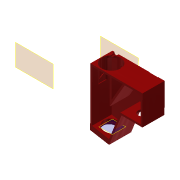
# Autodesk Inventor part: cellSTORM_v5_opticalstage
Saved by Autodesk Inventor 2022 (Build 260153000, 153)
## iProperties
Created: 2020-04-25
Part Number: cellSTORM_v5_opticalstage
Material: Generic
Document SubType Name: Modeling
Designer: diederichbenedict
Density: 1 g/cm^3
Appearance: Red
Author: diederichbenedict
Autodesk Inventor part; units mm, degrees
ref_plane "YZ Plane" through (0, 0, 0) normal (1, 0, 0) x (0, 1, 0)
ref_plane "XZ Plane" through (0, 0, 0) normal (0, 1, 0) x (-1, 0, 0)
ref_plane "XY Plane" through (0, 0, 0) normal (0, 0, 1) x (1, 0, 0)
ref_plane "Work Plane1" through (0, 0, 0) normal (0, 0, 1) x (1, 0, 0)
ref_plane "Work Plane2" through (79.8747, 18.9526, -58.9639) normal (0, 0.0044332, 0.9999902) x (1, 0, 0)
sketch "Sketch2" plane through (79.8747, 18.9526, -58.9639) normal (0, 0.0044332, 0.9999902) x (1, 0, 0)
  line L0 (-7.339, -43.0706) -> (-11.339, -43.0706)
  line L1 (-7.339, -43.0706) -> (-3.339, -43.0706) construction
  line L2 (-11.339, -43.0706) -> (-11.339, -85.3323)
  line L3 (-11.339, -85.3323) -> (19.5839, -90.7849)
  line L4 (39.661, -39.3323) -> (73.661, -39.3323)
  line L5 (-28.496, 8.6677) -> (-11.339, 8.6677)
  line L6 (-11.339, 8.6677) -> (-11.339, -43.0706)
  line L7 (19.5839, -90.7849) -> (39.661, -39.3323)
  line L8 (-28.496, 8.6677) -> (73.661, 8.6677)
  line L9 (73.661, 8.6677) -> (73.661, -39.3323)
  line L10 (-7.2559, -79.452) -> (-8.211, -84.8684)
  line L11 (17.7582, -83.8627) -> (16.8031, -89.2791)
  ellipse E0 centre (4.2527, -87.32) end of major axis (-8.0082, -85.158) minor radius 0.0544 projected
  line L12 (38.645, -66.6078) -> (38.645, -46.6079) projected
  ellipse E1 centre (54.8542, 5.5271) end of major axis (42.3472, 7.7324) minor radius 0.0554 projected
  point P0 (-79.8747, -19.2138)
  dimension "d0" = 4
  dimension "d1" = 180
  dimension "d156" = 3
  dimension "d157" = 3
  dimension "d158" = 1
  dimension "d159" = 94
  dimension "d160" = 85
  dimension "d161" = 48
  dimension "d163" = 34
  constraints: 24 end point, 4 horizontal, 2 collinear, 1 parallel, 1 perpendicular, 1 vertical, 9 other
  measures "d0" distance of L0.start L0.end
  measures "d1" angle of L0 L1
  measures "d156" distance from line of L2.end L10
  measures "d157" distance from line of L3.end L11
  measures "d158" distance from line of L3 L11.end
  measures "d159" distance from line of L8 L2.end
  measures "d160" distance between parallel lines of L9 L6
  measures "d161" distance between parallel lines of L8 L4
  measures "d163" distance from line of L9 L4.start
extrude "Extrusion1" add sketch "Sketch2" along normal blind 4 contours L6 L8 L9 L4 L7 L3 L2 | E0 | E1
sketch "Sketch3" plane through (79.8747, 18.9703, -54.964) normal (0, 0.0044332, 0.9999902) x (1, 0, 0)
  line L0 (73.661, 8.6677) -> (-11.339, 8.6677) projected
  line L1 (-11.339, 8.6677) -> (-11.339, -85.3323) projected
  line L2 (-11.339, -85.3323) -> (19.5839, -90.7849) projected
  line L3 (19.5839, -90.7849) -> (39.661, -39.3323) projected
  line L4 (39.661, -39.3323) -> (73.661, -39.3323) projected
  line L5 (73.661, -39.3323) -> (73.661, 8.6677) projected
  line L6 (70.661, 5.6677) -> (-8.339, 5.6677)
  line L7 (-8.339, 5.6677) -> (-8.339, -82.815)
  line L8 (-8.339, -82.815) -> (17.6831, -87.4034)
  line L9 (17.6831, -87.4034) -> (37.6113, -36.3323)
  line L10 (37.6113, -36.3323) -> (70.661, -36.3323)
  line L11 (70.661, -36.3323) -> (70.661, 5.6677)
  line L12 (20.3299, 5.6677) -> (20.3299, -36.4597)
  line L13 (20.3299, -36.4597) -> (44.6523, 5.6677)
  line L14 (41.1882, 5.6677) -> (23.3299, -25.2636)
  line L15 (23.3299, -25.2636) -> (23.3299, 5.6677)
  line L16 (50.5927, -0.5756) -> (7.6402, -74.9707)
  point P0 (-79.8747, -19.2138)
  point P1 (-36.2088, 5.0266)
  dimension "d165" = 3
  dimension "d166" = 3
  dimension "d167" = 3
  constraints: 22 end point, 4 point on line, 2 parallel, 1 perpendicular, 1 vertical, 8 other
  measures "d165" distance between parallel lines of L5 L11
  measures "d166" distance between parallel lines of L12 L15
  measures "d167" distance between parallel lines of L13 L14
extrude "Extrusion2" add sketch "Sketch3" along normal blind 32 contours L5 L4 L3 L2 L1 L0 | L13 L12 L6 L15 L14
ref_plane "Work Plane3" through (51.6835, -64.2382, -58.0722) normal (0.309017, 0.9510565, 0) x (-0.6726294, 0.2185505, 0.7069691)
ref_plane "Work Plane4" through (49.8294, -69.9446, -58.0722) normal (-0.309017, -0.9510565, 0) x (0.6723676, -0.2184655, 0.7072444)
sketch "Sketch7" plane through (51.6691, -60.199, -22.6127) normal (0.1736498, 0.9847978, -0.0043659) x (0.9848075, -0.1736481, 0.0007698)
  circle A0 centre (33.3557, 17.7195) radius 12
  ellipse E0 centre (33.3557, 17.7195) end of major axis (45.8057, 17.7195) minor radius 12.4499 projected
  point P0 (-61.3202, -22.8793)
  dimension "d33" = 24
  constraints: 1 centre point, 1 coincident
  measures "d33" diameter of A0
extrude "Extrusion5" cut sketch "Sketch7" against normal blind 5 contours A0
ref_plane "Work Plane5" through (122.0405, 25.1021, -58.0722) normal (-0.309017, -0.9510565, 0) x (0.6723676, -0.2184655, 0.7072444)
sketch "Sketch11" plane through (47.2299, 24.638, -54.9891) normal (0, 0.9999902, -0.0044332) x (1, 0, 0)
  circle A0 centre (37.785, -14.6472) radius 15.35
  ellipse E0 centre (37.785, -14.6472) end of major axis (51.685, -14.6472) minor radius 13.8999 projected
  point P0 (-47.2299, -54.8793)
  dimension "d43" = 30.7
  constraints: 1 centre point, 1 coincident
  measures "d43" diameter of A0
extrude "Extrusion9" cut sketch "Sketch11" along normal mid plane 60 contours A0 | E0
sketch "Sketch13" plane through (79.8747, 18.9703, -54.964) normal (0, 0.0044332, 0.9999902) x (1, 0, 0)
  line L0 (-33.2896, 17.9525) -> (-33.2896, -60.0475) construction
  line L1 (-28, 13.8293) -> (35.6078, 13.8293) construction
  line L2 (35.6078, 13.8293) -> (35.6078, 11.1076) construction
  line L3 (35.6078, 11.1076) -> (6.7488, -25.8302) construction
  line L4 (6.7488, -25.8302) -> (6.7488, 3.4793) construction
  line L5 (6.7488, 3.4793) -> (-28, 3.4793) construction
  line L6 (-28, 3.4793) -> (-28, 13.8293) construction
  line L7 (-29, -27.5207) -> (-29, -3.5207) construction
  line L8 (-0.2512, -3.5207) -> (-0.2512, -27.5207) projected
  line L9 (73.7104, 17.9525) -> (-33.2896, 17.9525) projected
  line L10 (73.7104, -38.0475) -> (73.7104, 17.9525) projected
  line L11 (-33.2896, -60.0475) -> (-4.8316, -73.3178) projected
  line L12 (-4.8316, -73.3178) -> (42.7104, -38.0475) projected
  line L13 (42.7104, -38.0475) -> (73.7104, -38.0475) projected
  point P0 (-79.8747, -19.2138)
  point P1 (-28, 13.8795)
  point P2 (2.2283, 13.8293)
  point P3 (27.2605, 13.8293)
  point P4 (24.4005, -3.237)
  point P5 (6.7488, -3.2707)
  point P6 (-4.2512, -23.8533)
  point P7 (-25, -23.8533)
  point P8 (-15.0063, 13.8293)
  point P9 (19.8117, 13.8293)
  point P10 (14.5771, -3.2707)
  point P11 (6.7488, -22.2564)
  dimension "d56" = 4
  dimension "d65" = 4
  constraints: 12 end point, 8 point on line, 1 coincident
  measures "d56" distance from line of point (-25, -23.853) L7
  measures "d65" distance from line of L8 point (-4.251, -23.853)
hole "Hole1" at (51.8747, 32.8497, -55.0255) at (82.103, 32.7995, -55.0253) at (107.1351, 32.7995, -55.0253) at (104.2752, 15.7334, -54.9496) at (86.6235, 15.6997, -54.9495) at (75.6235, -4.8827, -54.8582) at (54.8747, -4.8827, -54.8582) at (86.6235, -3.2858, -54.8653) at (94.4518, 15.6997, -54.9495) at (99.6864, 32.7995, -55.0253) at (64.8684, 32.7995, -55.0253) direction (0, -0.0044332, -0.9999902) diameter 2.9 depth 8 tip angle 118
ref_plane "Arbeitsebene11" through (104.1095, -44.1462, -23.1152) normal (0, -1, 0) x (1, 0, 0)
sketch "Sketch21" plane through (104.1095, -44.1462, -23.1152) normal (0, -1, 0) x (1, 0, 0)
  circle A0 centre (31.8151, -17.35) radius 7 projected
  point P0 (-104.1095, 23.1152)
extrude "Extrusion17" cut sketch "Sketch21" against normal blind 50
sketch "Sketch22" plane through (68.5356, -66.3788, -58.5856) normal (-1, 0, 0) x (0, 0.0044332, 0.9999902)
  line L0 (0, 94) -> (0, 0) projected
  line L1 (0, 0) -> (36, 0) projected
  line L2 (4, 109.1334) -> (4, 78) projected
  line L3 (4, 59.5268) -> (36, 59.5268) projected
  line L4 (4, 78) -> (36, 59.5268)
  line L5 (36, 59.5268) -> (4, 59.5268)
  line L6 (4, 78) -> (4, 0) projected
  line L7 (4, 59.5268) -> (4, 78)
  line L8 (36, 94) -> (36, 0) projected
  line L9 (0, 94) -> (36, 94) projected
  point P0 (58.8793, 66.1185)
  constraints: 6 end point, 1 perpendicular
extrude "Extrusion18" add sketch "Sketch22" against normal blind 2 contours L4 L3 L6
sketch "Sketch25" plane through (79.8747, 18.9526, -58.9639) normal (0, -0.0044332, -0.9999902) x (-1, 0, 0)
  line L0 (0.0762, 6.8793) -> (0.0762, 10.0793) projected
  line L1 (0.0762, 6.8793) -> (0.0762, 10.0793) projected
  point P0 (79.8747, -19.2138)
  point P1 (4.7512, 8.4793)
  point P2 (24.7512, 8.4793)
hole "Hole3" at (55.1235, 27.4318, -59.0015) at (75.1235, 27.4318, -59.0015) direction (0, 0.0044332, 0.9999902) diameter 3 depth 12 tip angle 118 counterbore diameter 7 counterbore depth 3
sketch "Skizze26" plane through (79.8747, 18.9526, -58.9639) normal (0, -0.0044332, -0.9999902) x (-1, 0, 0)
  circle A0 centre (-56.1499, 7.231) radius 1.75 projected
  circle A1 centre (-56.1499, -2.769) radius 1.75 projected
  circle A2 centre (-56.1499, -12.769) radius 1.75 projected
  circle A3 centre (-56.1499, -22.769) radius 1.75 projected
  point P0 (79.8747, -19.2138)
hole "Bohrung4" at (136.0246, 26.1835, -58.996) direction (0, 0.0044332, 0.9999902) diameter 2.8 depth 12 tip angle 118
pattern_linear "Rechteckige Anordnung1" count 12 spacing 12.5 along (0, -0.9999902, 0.0044332) of "Bohrung4"
sketch "Skizze28" plane through (79.8747, 18.9526, -58.9639) normal (0, -0.0044332, -0.9999902) x (-1, 0, 0)
  line L0 (-50.0499, -35.324) -> (-50.0499, -2.924) projected
  line L1 (-62.0499, -35.324) -> (-62.0499, -2.924) projected
  line L2 (-49.0499, 19.5051) -> (-63.0499, 19.5051)
  line L3 (-63.0499, 19.5051) -> (-63.0499, -40.5846)
  line L4 (-63.0499, -40.5846) -> (-49.0499, -40.5846)
  line L5 (-49.0499, -40.5846) -> (-49.0499, 19.5051)
  point P0 (79.8747, -19.2138)
  dimension "d134" = 1
  dimension "d135" = 1
  constraints: 8 end point, 2 parallel, 1 horizontal, 1 perpendicular
  measures "d134" distance between parallel lines of L0 L5
  measures "d135" distance between parallel lines of L3 L1
extrude "Extrusion21" cut sketch "Skizze28" against normal blind 0.5
sketch "Skizze30" plane through (71.5356, -63.8438, -54.5968) normal (0.1736498, 0.9847978, -0.0043659) x (0.9848075, -0.1736481, 0.0007698)
  circle A0 centre (13.1827, -14.2805) radius 12 projected
  line L0 (-2.5173, -32) -> (28.8827, -32) projected
  line L1 (27.1827, 3.439) -> (-0.8173, 3.439)
  line L2 (-0.8173, 3.439) -> (-0.8173, -32)
  line L3 (-0.8173, -32) -> (27.1827, -32)
  line L4 (27.1827, -32) -> (27.1827, 3.439)
  line L5 (27.1827, 3.439) -> (-0.8173, -32) construction
  line L6 (-0.8173, 3.439) -> (27.1827, -32) construction
  circle A1 centre (13.1827, -14.2805) radius 12.75
  point P0 (-81.4932, -54.8793)
  point P1 (27.1827, -32)
  dimension "d168" = 28
  dimension "d171" = 25.5
  constraints: 12 end point, 2 midpoint, 2 parallel, 1 centre point, 1 coincident, 1 horizontal, 1 perpendicular, 1 point on line
  measures "d168" distance of L3.end L2.end
  measures "d171" diameter of A1
extrude "Extrusion23" add sketch "Skizze30" along normal blind 5 contours L2 L1 L4 L0
body "Solid1"
